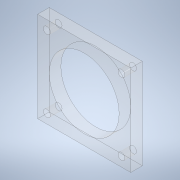
# Autodesk Inventor part: 103.016.01_Zwischenstueck_oben
Saved by Autodesk Inventor 2021 (Build 250183000, 183)
## iProperties
Created: 2021-11-25
Part Number: 103.016.01_Zwischenstueck_oben
Material: PMMA-Kunststoff
Document SubType Name: Modeling
Designer: Sebastian Seewald
Mass: 30.5736 g
Surface Area: 90.6063 cm^2
Volume: 25.7354 cm^3
Density: 1.188 g/cm^3
Appearance: Polycarbonat - klar
Author: Sebastian Seewald
Autodesk Inventor part; units mm, degrees
ref_plane "YZ Plane" through (0, 0, 0) normal (1, 0, 0) x (0, 1, 0)
ref_plane "XZ Plane" through (0, 0, 0) normal (0, 1, 0) x (-1, 0, 0)
ref_plane "XY Plane" through (0, 0, 0) normal (0, 0, 1) x (1, 0, 0)
sketch "Skizze1" plane through (0, 0, 0) normal (0, 0, 1) x (1, 0, 0)
  line L0 (0, 0) -> (60, 0)
  line L1 (60, 0) -> (60, 58.25)
  line L2 (60, 58.25) -> (0, 58.25)
  line L3 (0, 58.25) -> (0, 0)
  circle A0 centre (6, 52.25) radius 2.25
  circle A1 centre (54, 52.25) radius 2.25
  circle A2 centre (54, 6) radius 2.25
  circle A3 centre (6, 6) radius 2.25
  dimension "d0" = 60
  dimension "d1" = 58.25
  dimension "d2" = 4.5
  dimension "d3" = 4.5
  dimension "d4" = 4.5
  dimension "d5" = 4.5
  dimension "d6" = 48
  dimension "d7" = 46.25
  dimension "d8" = 6
  dimension "d9" = 6
  dimension "d10" = 6
  dimension "d11" = 6
  constraints: 8 end point, 4 centre point, 2 horizontal alignment, 2 parallel, 2 vertical alignment, 1 horizontal, 1 perpendicular
  measures "d0" distance of L1.end L2.end
  measures "d1" distance of L0.end L1.end
  measures "d2" diameter of A0
  measures "d3" diameter of A1
  measures "d4" diameter of A2
  measures "d5" diameter of A3
  measures "d6" distance of A1.centre A0.centre
  measures "d7" distance of A0.centre A3.centre
  measures "d8" distance from line of L2 A0.centre
  measures "d9" distance from line of L3 A0.centre
  measures "d10" distance from line of L0 A3.centre
  measures "d11" distance from line of L3 A3.centre
extrude "Extrusion1" add sketch "Skizze1" along normal blind 7.5
sketch "Skizze2" plane through (0, 0, 7.5) normal (0, 0, 1) x (1, 0, 0)
  circle A0 centre (30, 29.125) radius 22.5
  line L0 (60, 58.25) -> (0, 58.25) projected
  line L1 (0, 58.25) -> (0, 0) projected
  dimension "d14" = 45
  dimension "d15" = 29.125
  dimension "d16" = 30
  constraints: 1 centre point
  measures "d14" diameter of A0
  measures "d15" distance from line of L0 A0.centre
  measures "d16" distance from line of L1 A0.centre
extrude "Extrusion2" cut sketch "Skizze2" against normal blind 10
